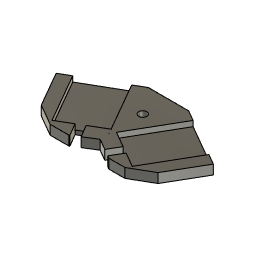
Deckenbefestigung-platte v2 (Autodesk Fusion 360 design; units mm, degrees)
Autodesk Fusion 360 part; units mm, degrees
sketch "Skizze1" plane through (0, 0, 0) normal (0, 0, 1) x (1, 0, 0)
  line L0 (0.0185, 31.9947) -> (0.0278, 32)
  line L1 (-1.9679, 35.4635) -> (-7.7548, 45.5067)
  line L2 (-29.6959, 19.4899) -> (-35.4814, 29.5308)
  line L3 (-43.2796, 25.0376) -> (-27.6989, 16.024)
  line L4 (-0.7462, 33.3433) -> (0.0278, 32)
  line L5 (0.0278, 32) -> (0.8041, 33.3419)
  line L6 (0.0093, 16) -> (-27.6989, 16.024)
  line L7 (-7.7548, 45.5067) -> (-22.7322, 71.5005)
  line L8 (-35.4814, 29.5308) -> (-50.4589, 55.5246)
  line L9 (-22.7322, 71.5005) -> (-50.4589, 55.5246)
  line L10 (-22.7322, 71.5005) -> (-14.9341, 75.9937)
  line L11 (-43.2796, 25.0376) -> (-58.257, 51.0313)
  line L12 (-50.4589, 55.5246) -> (-58.257, 51.0313)
  line L13 (0.0434, 74.9415) -> (0, 0)
  line L14 (35.5156, 29.4897) -> (50.5231, 55.4661)
  line L15 (22.815, 71.4741) -> (15.022, 75.9764)
  line L16 (0.0093, 16) -> (27.7175, 15.992)
  line L17 (7.8074, 45.4977) -> (22.815, 71.4741)
  line L18 (29.7185, 19.4555) -> (35.5156, 29.4897)
  line L19 (43.3085, 24.9874) -> (27.7175, 15.992)
  line L20 (50.5231, 55.4661) -> (58.3161, 50.9638)
  line L21 (22.815, 71.4741) -> (50.5231, 55.4661)
  line L22 (43.3085, 24.9874) -> (58.3161, 50.9638)
  line L23 (2.0103, 35.4635) -> (7.8074, 45.4977)
  line L24 (15.022, 75.9764) -> (-14.9341, 75.9937)
  line L25 (29.7185, 19.4555) -> (2.0103, 35.4635)
  line L26 (-29.6959, 19.4899) -> (-29.2073, 19.4555)
  line L27 (-29.2073, 19.4555) -> (-1.9679, 35.4635)
  line L28 (0.0185, 31.9947) -> (0.0093, 32)
  line L29 (0.0434, 50) -> (0.029, 50.025)
  line L30 (0.0145, 50) -> (0.029, 50.025)
  line L31 (-29.2073, 19.4555) -> (-29.5555, 19.2509)
  line L32 (-29.6959, 19.4899) -> (-29.5555, 19.2509)
  dimension "d1" = 50
  dimension "d2" = 32
  dimension "d8" = 30
  dimension "d10" = 30
  constraint coincident L13.end origin
  constraint perpendicular L0 L4
  constraint perpendicular L8 L9
  constraint perpendicular L7 L10
  constraint perpendicular L10 L29
  constraint perpendicular L11 L12
  constraint coincident L13 L6.start
  constraint symmetric L29.start L13 L30.start
  constraint symmetric L3.start L13 L19.start
  constraint symmetric L3.end L13 L16.end
  constraint symmetric L0.end L13 L28.end
  constraint symmetric L1.end L13 L17.start
  constraint symmetric L2.end L13 L14.start
  constraint symmetric L7.end L13 L15.start
  constraint symmetric L8.end L13 L14.end
  constraint symmetric L10.end L13 L15.end
  constraint symmetric L11.end L13 L20.end
  constraint symmetric L13 L6.start L16.start
  constraint perpendicular L23 L25
  constraint coincident L13 L29.end
  constraint parallel L27 L31
  constraint perpendicular L31 L32
  measures "d1" distance of L29.start L13.end
  measures "d2" distance of L3.end L0.end
  measures "d8" distance of L1.end L7.end
  measures "d10" distance of L3.start L11.end
extrude "Extrusion3" add sketch "Skizze1" along normal blind 4 contours L1 L2 L3 L6 L7 L8 L10 L11 L12 L14 L15 L16 L17 L18 L19 L20 L22 L23 L24 L25 L27 L31 L32
extrude "Extrusion4" add sketch "Skizze1" along normal blind 3 contours L1 L2 L7 L8 L9 L26 L27 | L14 L17 L18 L21 L23 L25
extrude "Extrusion5" add 1 faces at (0.6994, 62.4779, 4) along direction (0, 0, 1) blind 3
hole "Bohrung1" at (0.0504, 56.8999, 7) direction (0, 0, -1) diameter 6 depth 8 tip angle 118
sketch "Skizze2" plane through (0, 0, 7) normal (0, 0, 1) x (-1, 0, 0)
  circle A0 centre (-0.0504, -56.8999) radius 3
  line L0 (-0.0278, -32) -> (-0.0185, -31.9947)
  line L1 (-0.0185, -31.9947) -> (-0.0185, -32.016)
  line L2 (-0.0185, -32.016) -> (-0.0278, -32)
  line L3 (29.6959, -19.4899) -> (50.4589, -55.5246)
  line L4 (50.4589, -55.5246) -> (58.257, -51.0313)
  line L5 (58.257, -51.0313) -> (43.2796, -25.0376)
  line L6 (43.2796, -25.0376) -> (27.6989, -16.024)
  line L7 (27.6989, -16.024) -> (-0.0093, -16)
  line L8 (-0.0093, -16) -> (-27.7175, -15.992)
  line L9 (-27.7175, -15.992) -> (-43.3085, -24.9874)
  line L10 (-43.3085, -24.9874) -> (-58.3161, -50.9638)
  line L11 (-58.3161, -50.9638) -> (-50.5231, -55.4661)
  line L12 (-50.5231, -55.4661) -> (-29.7185, -19.4555)
  line L13 (-29.7185, -19.4555) -> (-2.0103, -35.4635)
  line L14 (-2.0103, -35.4635) -> (-22.815, -71.4741)
  line L15 (-22.815, -71.4741) -> (-15.022, -75.9764)
  line L16 (-15.022, -75.9764) -> (14.9341, -75.9937)
  line L17 (14.9341, -75.9937) -> (22.7322, -71.5005)
  line L18 (22.7322, -71.5005) -> (1.9679, -35.4635)
  line L19 (1.9679, -35.4635) -> (29.5555, -19.2509)
  line L20 (29.5555, -19.2509) -> (29.6959, -19.4899)
  line L21 (-15.8644, -15.9954) -> (-0.4521, -24.8996)
  line L22 (13.8448, -16.012) -> (-0.4521, -24.8996)
  constraint coincident L8 L21.start
  constraint parallel L13 L21
  constraint midpoint L7 L22.start
extrude "Extrusion6" cut sketch "Skizze2" against normal blind 23 contours L7 L8 L21 L22
sketch "Skizze3" plane through (0, 0, 3) normal (0, 0, 1) x (-1, 0, 0)
  line L0 (29.6959, -19.4899) -> (29.2073, -19.4555)
  line L1 (29.2073, -19.4555) -> (1.9679, -35.4635)
  line L2 (1.9679, -35.4635) -> (22.7322, -71.5005)
  line L3 (22.7322, -71.5005) -> (50.4589, -55.5246)
  line L4 (50.4589, -55.5246) -> (29.6959, -19.4899)
  line L5 (18.7813, -25.5826) -> (13.6085, -28.6226)
  line L6 (18.7813, -25.5826) -> (13.1225, -15.9535)
  line L7 (13.6085, -28.6226) -> (7.9138, -18.9326)
  line L8 (7.9138, -18.9326) -> (13.1225, -15.9535)
  line L9 (-0.0434, -74.9415) -> (0, 0)
  line L10 (-13.6416, -28.6068) -> (-7.9358, -18.9234)
  line L11 (-7.9358, -18.9234) -> (-13.1409, -15.9383)
  line L12 (-18.8109, -25.5609) -> (-13.1409, -15.9383)
  line L13 (-18.8109, -25.5609) -> (-13.6416, -28.6068)
  dimension "d23" = 6
  dimension "d24" = 12.5
  constraint coincident L1 L5.start
  constraint perpendicular L5 L6
  constraint perpendicular L1 L7
  constraint symmetric L5.start L9 L12.start
  constraint symmetric L5.end L9 L10.start
  constraint symmetric L6.end L9 L11.end
  constraint symmetric L7.end L9 L10.end
  measures "d23" distance of L5.start L5.end
  measures "d24" distance of L0.start L5.start
extrude "Extrusion7" cut sketch "Skizze3" along normal mid plane 26 contours L1 L5 L6 L7 L8 | L10 L11 L12 L13
extrude "Extrusion8" cut 1 faces at (17.0878, 26.5762, 2.3333) along direction (0.507661, 0.861557, 0) blind 0.5
